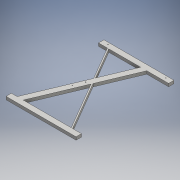
# Autodesk Inventor part: Desk stand
Saved by Autodesk Inventor 2016 (Build 200138000, 138)
## iProperties
Created: 2015-11-19
Part Number: Desk stand
Material: 常规
Document SubType Name: Modeling
Designer: Shawn Shi Feng
Density: 1 g/cm^3
Appearance: 默认
Author: Shawn Shi Feng
Autodesk Inventor part; units mm, degrees
ref_plane "YZ Plane" through (0, 0, 0) normal (1, 0, 0) x (0, 1, 0)
ref_plane "XZ Plane" through (0, 0, 0) normal (0, 1, 0) x (-1, 0, 0)
ref_plane "XY Plane" through (0, 0, 0) normal (0, 0, 1) x (1, 0, 0)
sketch "草图1" plane through (0, 0, 0) normal (0, 0, 1) x (1, 0, 0)
  line L0 (-510.4235, -20.2532) -> (9.5765, -20.2532)
  line L1 (9.5765, -20.2532) -> (9.5765, -60.2532)
  line L2 (9.5765, -60.2532) -> (-510.4235, -60.2532)
  line L3 (-510.4235, -60.2532) -> (-510.4235, -20.2532)
  line L4 (-510.4235, -707.2532) -> (9.5765, -707.2532)
  line L5 (9.5765, -707.2532) -> (9.5765, -747.2532)
  line L6 (9.5765, -747.2532) -> (-510.4235, -747.2532)
  line L7 (-510.4235, -747.2532) -> (-510.4235, -707.2532)
  line L8 (-66.4235, -707.2532) -> (-274.0901, -351.8026)
  line L9 (-56.4235, -707.2532) -> (-269.9235, -341.818)
  line L10 (-296.1735, -296.8875) -> (-434.4235, -60.2532)
  line L11 (-300.3401, -306.872) -> (-444.4235, -60.2532)
  line L12 (-152.4235, -60.2532) -> (-269.9235, -341.818)
  line L13 (-274.0901, -351.8026) -> (-422.4235, -707.2532)
  line L14 (-467.4235, -707.2532) -> (-300.3401, -306.872)
  line L15 (-296.1735, -296.8875) -> (-197.4235, -60.2532)
  point P0 (0, 0)
  dimension "d0" = 520
  dimension "d1" = 40
  dimension "d2" = 162
  dimension "d3" = 45
  dimension "d4" = 647
  dimension "d5" = 40
  dimension "d6" = 43
  dimension "d7" = 66
  dimension "d8" = 66
  dimension "d9" = 10
  constraints: 32 end point, 12 parallel, 8 point on line, 2 horizontal, 2 perpendicular
  measures "d0" distance of L0.start L0.end
  measures "d1" distance of L0.end L1.end
  measures "d2" distance of L1.end L12.start
  measures "d3" distance of L12.start L15.end
  measures "d4" distance between parallel lines of L4 L2
  measures "d5" distance of L4.end L5.end
  measures "d6" distance of L14.start L4.start
  measures "d7" distance of L4.end L9.start
  measures "d8" distance of L11.end L2.end
  measures "d9" distance of L8.start L9.start
extrude "拉伸1" add sketch "草图1" along normal blind 22 contours L0 L1 L2 L3 | L2 L10 L15 L12 L9 L4 L8 L13 L14 L11 | L4 L5 L6 L7
sketch "草图2" plane through (0, 0, 22) normal (0, 0, 1) x (1, 0, 0)
  line L0 (9.5765, -60.2532) -> (9.5765, -20.2532) projected
  circle A0 centre (-35.4235, -35.2532) radius 2.5
  line L1 (9.5765, -20.2532) -> (-510.4235, -20.2532) projected
  line L2 (-510.4235, -20.2532) -> (-510.4235, -60.2532) projected
  circle A1 centre (-465.4235, -35.2532) radius 2.5
  line L3 (-300.3401, -306.872) -> (-467.4235, -707.2532) projected
  circle A2 centre (-306.5264, -360.6449) radius 2.5
  circle A3 centre (-335.4105, -429.8598) radius 2.5
  point P0 (0, 0)
  dimension "d12" = 45
  dimension "d13" = 5
  dimension "d14" = 15
  dimension "d15" = 45
  dimension "d16" = 15
  dimension "d17" = 5
  dimension "d46" = 5
  dimension "d47" = 5
  dimension "d48" = 75
  constraints: 4 centre point, 4 coincident
  measures "d12" distance from line of L0 point (-35.423, -35.253)
  measures "d13" diameter of A0
  measures "d14" distance from line of L1 point (-35.423, -35.253)
  measures "d15" distance from line of L2 point (-465.423, -35.253)
  measures "d16" distance from line of point (-465.423, -35.253) L1
  measures "d17" diameter of A1
  measures "d46" diameter of A2
  measures "d47" diameter of A3
  measures "d48" distance of point (-306.526, -360.645) point (-335.411, -429.86)
extrude "拉伸2" cut sketch "草图2" against normal blind 25
thread "螺纹1" size "M5x0.8" class "6H" standard "ANSI Metric M Profile" full length
thread "螺纹2" size "M5x0.8" class "6H" standard "ANSI Metric M Profile" full length
